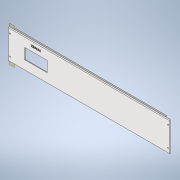
# Autodesk Inventor part: Case_Back
Saved by Autodesk Inventor 2022.2 (Build 262287010, 287A)
## iProperties
Created: 2024-11-06
Part Number: Case_Back
Material: Generisch
Document SubType Name: Modeling
Designer: ppovolni
Density: 1 g/cm^3
Appearance: Vorgabe
Author: ppovolni
Autodesk Inventor part; units mm, degrees
ref_plane "YZ Plane" through (0, 0, 0) normal (1, 0, 0) x (0, 1, 0)
ref_plane "XZ Plane" through (0, 0, 0) normal (0, 1, 0) x (-1, 0, 0)
ref_plane "XY Plane" through (0, 0, 0) normal (0, 0, 1) x (1, 0, 0)
ref_plane "Arbeitsebene1" through (-412.466, 0, 0) normal (0, 0, 1) x (-1, 0, 0)
sketch "Skizze1" plane through (-412.466, 0, 0) normal (0, 0, 1) x (-1, 0, 0)
  line L0 (6.25, 41.6) -> (6.25, -41.6) projected
  line L1 (-418.716, -41.6) -> (-418.716, 41.6) projected
  circle A0 centre (-414.916, -26.5) radius 1.6 projected
  circle A1 centre (-414.916, 26.5) radius 1.6 projected
  circle A2 centre (2.45, -26.5) radius 1.6 projected
  circle A3 centre (2.45, 26.5) radius 1.6 projected
  line L2 (6.25, -39.7) -> (-418.716, -39.7)
  line L3 (6.25, 39.2) -> (-418.716, 39.2)
  line L4 (-406.216, -39.7) -> (-411.416, -39.7) construction
  line L5 (-411.416, 39.2) -> (-406.216, 39.2) construction
  line L6 (-6.25, -39.2) -> (-6.25, 39.7) construction
  line L7 (-406.216, 39.2) -> (-406.216, -39.7) construction
  point P0 (-412.466, 0)
  constraints: 4 end point, 4 point on line, 2 collinear, 2 horizontal
extrude "Extrusion1" add sketch "Skizze1" along normal blind 2
sketch "Skizze2" plane through (-412.466, 0, 2) normal (0, 0, 1) x (1, 0, 0)
  line L0 (36.25, 14.25) -> (95.75, 14.25)
  line L1 (95.75, 14.25) -> (95.75, -14.25)
  line L2 (95.75, -14.25) -> (36.25, -14.25)
  line L3 (36.25, -14.25) -> (36.25, 14.25)
  line L4 (6.25, 39.2) -> (6.25, -39.7) construction
  line L5 (36.25, 0) -> (95.75, 0) construction
  line L6 (36.25, 14.25) -> (95.75, 14.25) construction
  line L7 (36.25, 24.25) -> (36.25, 14.25) construction
  point P0 (412.466, 0)
  dimension "d2" = 28.5
  dimension "d3" = 59.5
  dimension "d4" = 30
  constraints: 14 end point, 2 horizontal, 2 midpoint, 2 parallel, 1 perpendicular, 1 point on line
  measures "d2" distance of L2.end L0.start
  measures "d3" distance of L0.start L0.end
  measures "d4" distance between parallel lines of L4 L3
extrude "Extrusion2" cut sketch "Skizze2" against normal up to surface (2 mm away)
sketch "Skizze3" plane through (-412.466, 0, 2) normal (0, 0, 1) x (1, 0, 0)
  line L0 (36.25, 14.25) -> (95.75, 14.25) construction
  line L1 (36.25, 14.25) -> (95.75, 14.25) construction
  line L2 (95.75, 14.25) -> (95.75, 24.25) construction
  line L3 (95.75, 24.25) -> (36.25, 24.25) construction
  line L4 (36.25, 24.25) -> (36.25, 14.25) construction
  line L5 (56.6422, 24.25) -> (52.9672, 24.25)
  line L6 (52.9672, 24.25) -> (52.9672, 25.0644)
  spline S0 degree 2 poles (52.9672, 25.0644) (53.4331, 25.4372) (54.1787, 26.0936) (54.4583, 26.3894) knots 0 0 0 1 2 2 2
  spline S1 degree 2 poles (54.4583, 26.3894) (54.827, 26.7743) (55.1552, 27.3618) (55.1552, 27.6698) knots 0 0 0 1 2 2 2
  spline S2 degree 2 poles (55.1552, 27.6698) (55.1552, 28.0182) (54.7378, 28.391) (54.3651, 28.391) knots 0 0 0 1 2 2 2
  spline S3 degree 2 poles (54.3651, 28.391) (54.1746, 28.391) (53.8343, 28.2978) (53.66, 28.2249) knots 0 0 0 1 2 2 2
  spline S4 degree 2 poles (53.66, 28.2249) (53.4899, 28.1479) (53.2468, 27.9858) (53.186, 27.9453) knots 0 0 0 1 2 2 2
  line L7 (53.186, 27.9453) -> (53.0887, 27.9453)
  line L8 (53.0887, 27.9453) -> (53.0887, 29.0353)
  spline S5 degree 2 poles (53.0887, 29.0353) (53.2994, 29.1365) (54.1989, 29.3472) (54.6163, 29.3472) knots 0 0 0 1 2 2 2
  spline S6 degree 2 poles (54.6163, 29.3472) (55.5077, 29.3472) (56.4234, 28.5531) (56.4234, 27.8359) knots 0 0 0 1 2 2 2
  spline S7 degree 2 poles (56.4234, 27.8359) (56.4234, 27.3942) (56.0061, 26.5434) (55.5239, 26.0571) knots 0 0 0 1 2 2 2
  spline S8 degree 2 poles (55.5239, 26.0571) (55.22, 25.7573) (54.6487, 25.2913) (54.5231, 25.1941) knots 0 0 0 1 2 2 2
  line L9 (54.5231, 25.1941) -> (56.6422, 25.1941)
  line L10 (56.6422, 25.1941) -> (56.6422, 24.25)
  spline S9 degree 2 poles (60.8967, 25.7654) (60.8967, 25.3967) (60.6252, 24.7929) (60.3618, 24.5823) knots 0 0 0 1 2 2 2
  spline S10 degree 2 poles (60.3618, 24.5823) (60.0985, 24.3716) (59.3813, 24.1447) (58.8667, 24.1447) knots 0 0 0 1 2 2 2
  spline S11 degree 2 poles (58.8667, 24.1447) (58.2832, 24.1447) (57.4485, 24.3391) (57.1852, 24.4607) knots 0 0 0 1 2 2 2
  line L11 (57.1852, 24.4607) -> (57.1852, 25.5466)
  line L12 (57.1852, 25.5466) -> (57.3067, 25.5466)
  spline S12 degree 2 poles (57.3067, 25.5466) (57.5823, 25.3724) (58.3237, 25.113) (58.6317, 25.113) knots 0 0 0 1 2 2 2
  spline S13 degree 2 poles (58.6317, 25.113) (58.814, 25.113) (59.2395, 25.1779) (59.3853, 25.2832) knots 0 0 0 1 2 2 2
  spline S14 degree 2 poles (59.3853, 25.2832) (59.4988, 25.3683) (59.6365, 25.6155) (59.6365, 25.8383) knots 0 0 0 1 2 2 2
  spline S15 degree 2 poles (59.6365, 25.8383) (59.6365, 26.0612) (59.4421, 26.3002) (59.28, 26.357) knots 0 0 0 1 2 2 2
  spline S16 degree 2 poles (59.28, 26.357) (59.1179, 26.4137) (58.6682, 26.4259) (58.4939, 26.4259) knots 0 0 0 1 2 2 2
  line L13 (58.4939, 26.4259) -> (58.2792, 26.4259)
  line L14 (58.2792, 26.4259) -> (58.2792, 27.3051)
  line L15 (58.2792, 27.3051) -> (58.4777, 27.3051)
  spline S17 degree 2 poles (58.4777, 27.3051) (58.7046, 27.3051) (59.0895, 27.3456) (59.2233, 27.4064) knots 0 0 0 1 2 2 2
  spline S18 degree 2 poles (59.2233, 27.4064) (59.357, 27.4712) (59.5069, 27.6981) (59.5069, 27.8926) knots 0 0 0 1 2 2 2
  spline S19 degree 2 poles (59.5069, 27.8926) (59.5069, 28.0466) (59.3651, 28.237) (59.2638, 28.2897) knots 0 0 0 1 2 2 2
  spline S20 degree 2 poles (59.2638, 28.2897) (59.1422, 28.3505) (58.8181, 28.391) (58.7046, 28.391) knots 0 0 0 1 2 2 2
  spline S21 degree 2 poles (58.7046, 28.391) (58.5223, 28.391) (58.1374, 28.3059) (57.9591, 28.237) knots 0 0 0 1 2 2 2
  spline S22 degree 2 poles (57.9591, 28.237) (57.8173, 28.1844) (57.5093, 28.0142) (57.4364, 27.9696) knots 0 0 0 1 2 2 2
  line L16 (57.4364, 27.9696) -> (57.331, 27.9696)
  line L17 (57.331, 27.9696) -> (57.331, 29.0393)
  spline S23 degree 2 poles (57.331, 29.0393) (57.5904, 29.1487) (58.4656, 29.3553) (58.9234, 29.3553) knots 0 0 0 1 2 2 2
  spline S24 degree 2 poles (58.9234, 29.3553) (59.3691, 29.3553) (60.0255, 29.2014) (60.2565, 29.0515) knots 0 0 0 1 2 2 2
  spline S25 degree 2 poles (60.2565, 29.0515) (60.5118, 28.8934) (60.767, 28.4072) (60.767, 28.1033) knots 0 0 0 1 2 2 2
  spline S26 degree 2 poles (60.767, 28.1033) (60.767, 27.6738) (60.2727, 27.0336) (59.8675, 26.9404) knots 0 0 0 1 2 2 2
  line L18 (59.8675, 26.9404) -> (59.8675, 26.8918)
  spline S27 degree 2 poles (59.8675, 26.8918) (60.0458, 26.8675) (60.3861, 26.7378) (60.5482, 26.592) knots 0 0 0 1 2 2 2
  spline S28 degree 2 poles (60.5482, 26.592) (60.6981, 26.4623) (60.8967, 26.049) (60.8967, 25.7654) knots 0 0 0 1 2 2 2
  spline S29 degree 2 poles (65.3375, 26.75) (65.3375, 26.1017) (65.1309, 25.1293) (64.8999, 24.8011) knots 0 0 0 1 2 2 2
  spline S30 degree 2 poles (64.8999, 24.8011) (64.673, 24.4769) (63.9396, 24.1447) (63.4129, 24.1447) knots 0 0 0 1 2 2 2
  spline S31 degree 2 poles (63.4129, 24.1447) (62.8821, 24.1447) (62.1528, 24.4769) (61.9218, 24.8092) knots 0 0 0 1 2 2 2
  spline S32 degree 2 poles (61.9218, 24.8092) (61.6908, 25.1374) (61.4842, 26.1017) (61.4842, 26.75) knots 0 0 0 1 2 2 2
  spline S33 degree 2 poles (61.4842, 26.75) (61.4842, 27.4145) (61.6908, 28.3545) (61.9259, 28.6949) knots 0 0 0 1 2 2 2
  spline S34 degree 2 poles (61.9259, 28.6949) (62.1609, 29.0271) (62.9024, 29.3513) (63.4129, 29.3513) knots 0 0 0 1 2 2 2
  spline S35 degree 2 poles (63.4129, 29.3513) (63.9518, 29.3513) (64.673, 29.0109) (64.904, 28.6746) knots 0 0 0 1 2 2 2
  spline S36 degree 2 poles (64.904, 28.6746) (65.1309, 28.3464) (65.3375, 27.378) (65.3375, 26.75) knots 0 0 0 1 2 2 2
  spline S37 degree 2 poles (64.0774, 26.75) (64.0774, 27.6779) (63.7735, 28.4275) (63.4129, 28.4275) knots 0 0 0 1 2 2 2
  spline S38 degree 2 poles (63.4129, 28.4275) (63.0523, 28.4275) (62.7443, 27.6779) (62.7443, 26.7459) knots 0 0 0 1 2 2 2
  spline S39 degree 2 poles (62.7443, 26.7459) (62.7443, 25.8302) (63.0523, 25.0685) (63.4129, 25.0685) knots 0 0 0 1 2 2 2
  spline S40 degree 2 poles (63.4129, 25.0685) (63.7694, 25.0685) (64.0774, 25.8302) (64.0774, 26.75) knots 0 0 0 1 2 2 2
  line L19 (70.293, 29.25) -> (68.575, 24.25)
  line L20 (68.575, 24.25) -> (67.2662, 24.25)
  line L21 (67.2662, 24.25) -> (65.5482, 29.25)
  line L22 (65.5482, 29.25) -> (66.8489, 29.25)
  line L23 (66.8489, 29.25) -> (67.9388, 25.8586)
  line L24 (67.9388, 25.8586) -> (69.0247, 29.25)
  line L25 (69.0247, 29.25) -> (70.293, 29.25)
  line L26 (70.3254, 24.25) -> (72.015, 29.25)
  line L27 (72.015, 29.25) -> (73.3845, 29.25)
  line L28 (73.3845, 29.25) -> (75.0741, 24.25)
  line L29 (75.0741, 24.25) -> (73.7816, 24.25)
  line L30 (73.7816, 24.25) -> (73.4696, 25.2711)
  line L31 (73.4696, 25.2711) -> (71.8975, 25.2711)
  line L32 (71.8975, 25.2711) -> (71.5814, 24.25)
  line L33 (71.5814, 24.25) -> (70.3254, 24.25)
  line L34 (73.1941, 26.1787) -> (72.6836, 27.8318)
  line L35 (72.6836, 27.8318) -> (72.169, 26.1787)
  line L36 (72.169, 26.1787) -> (73.1941, 26.1787)
  spline S41 degree 2 poles (77.7686, 24.1528) (76.6422, 24.1528) (75.3213, 25.5142) (75.3213, 26.7459) knots 0 0 0 1 2 2 2
  spline S42 degree 2 poles (75.3213, 26.7459) (75.3213, 27.9331) (76.6463, 29.3472) (77.7727, 29.3472) knots 0 0 0 1 2 2 2
  spline S43 degree 2 poles (77.7727, 29.3472) (78.0685, 29.3472) (78.5466, 29.2784) (78.7654, 29.2216) knots 0 0 0 1 2 2 2
  spline S44 degree 2 poles (78.7654, 29.2216) (78.9356, 29.169) (79.3367, 28.9947) (79.4623, 28.9299) knots 0 0 0 1 2 2 2
  line L37 (79.4623, 28.9299) -> (79.4623, 27.7387)
  line L38 (79.4623, 27.7387) -> (79.3367, 27.7387)
  spline S45 degree 2 poles (79.3367, 27.7387) (79.2435, 27.8197) (78.968, 28.0466) (78.7938, 28.1519) knots 0 0 0 1 2 2 2
  spline S46 degree 2 poles (78.7938, 28.1519) (78.6195, 28.2613) (78.2022, 28.4113) (77.9712, 28.4113) knots 0 0 0 1 2 2 2
  spline S47 degree 2 poles (77.9712, 28.4113) (77.6998, 28.4113) (77.25, 28.2411) (77.0434, 28.0263) knots 0 0 0 1 2 2 2
  spline S48 degree 2 poles (77.0434, 28.0263) (76.857, 27.8359) (76.6179, 27.1835) (76.6179, 26.7419) knots 0 0 0 1 2 2 2
  spline S49 degree 2 poles (76.6179, 26.7419) (76.6179, 26.2759) (76.8651, 25.6398) (77.0677, 25.4453) knots 0 0 0 1 2 2 2
  spline S50 degree 2 poles (77.0677, 25.4453) (77.2622, 25.2549) (77.7403, 25.0887) (77.9793, 25.0887) knots 0 0 0 1 2 2 2
  spline S51 degree 2 poles (77.9793, 25.0887) (78.2265, 25.0887) (78.6763, 25.2549) (78.8302, 25.3562) knots 0 0 0 1 2 2 2
  spline S52 degree 2 poles (78.8302, 25.3562) (79.0004, 25.4575) (79.2557, 25.6722) (79.3489, 25.7573) knots 0 0 0 1 2 2 2
  line L39 (79.3489, 25.7573) -> (79.4623, 25.7573)
  line L40 (79.4623, 25.7573) -> (79.4623, 24.5823)
  spline S53 degree 2 poles (79.4623, 24.5823) (79.3246, 24.5174) (78.9639, 24.3553) (78.7694, 24.2986) knots 0 0 0 1 2 2 2
  spline S54 degree 2 poles (78.7694, 24.2986) (78.5344, 24.2257) (78.1252, 24.1528) (77.7686, 24.1528) knots 0 0 0 1 2 2 2
  point P0 (412.466, 0)
  dimension "d8" = 10
  constraints: 8 end point, 2 horizontal, 2 parallel, 1 perpendicular, 1 point on line
  measures "d8" distance of L1.end L2.end
extrude "Extrusion3" cut sketch "Skizze3" against normal blind 0.5
sketch "Skizze4" plane through (-412.466, 0, 0) normal (0, 0, -1) x (-1, 0, 0)
  line L0 (-406.216, -39.2) -> (-406.216, 39.7) construction
  line L1 (-6.25, 39.2) -> (-6.25, -39.7) construction
  line L2 (-418.716, 39.7) -> (6.25, 39.7) projected
  line L3 (6.25, -39.2) -> (-418.716, -39.2) projected
  line L4 (-405.216, 39.7) -> (-7.25, 39.7)
  line L5 (-7.25, 39.7) -> (-7.25, 37.7)
  line L6 (-7.25, 37.7) -> (-405.216, 37.7)
  line L7 (-405.216, 37.7) -> (-405.216, 39.7)
  line L8 (-405.216, -39.2) -> (-7.25, -39.2)
  line L9 (-7.25, -39.2) -> (-7.25, -37.2)
  line L10 (-7.25, -37.2) -> (-405.216, -37.2)
  line L11 (-405.216, -37.2) -> (-405.216, -39.2)
  point P0 (-412.466, 0)
  point P1 (-7.25, 38.7)
  point P2 (-405.216, 38.7)
  point P3 (-7.25, -38.2)
  point P4 (-7.25, -39.2)
  dimension "d11" = 2
  dimension "d12" = 1
  dimension "d13" = 1
  dimension "d14" = 2
  dimension "d15" = 1
  dimension "d16" = 1
  constraints: 16 end point, 4 parallel, 3 midpoint, 2 horizontal, 2 perpendicular, 2 point on line
  measures "d11" distance between parallel lines of L6 L2
  measures "d12" distance from line of point (-7.25, 38.7) L1
  measures "d13" distance from line of L0 point (-405.216, 38.7)
  measures "d14" distance between parallel lines of L3 L10
  measures "d15" distance between parallel lines of L0 L11
  measures "d16" distance from line of point (-7.25, -38.2) L1
extrude "Extrusion4" add sketch "Skizze4" along normal blind 4
fillet "Rundung1" radius 2 4 edges at (-206.233, 39.7, 2) (-206.233, -39.2, 2) (-206.233, -37.2, 0) (-206.233, 37.7, 0)
